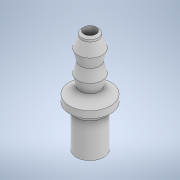
# Autodesk Inventor part: Thread to Barbed 3-32 inch and 10-32 hole
Saved by Autodesk Inventor 2021 (Build 250183000, 183)
## iProperties
Created: 2020-12-17
Part Number: Thread to Barbed 3-32 inch and 10-32 hole
Material: Generic
Document SubType Name: Modeling
Designer: natha
Density: 1 g/cm^3
Appearance: Default
Author: natha
Autodesk Inventor part; units mm, degrees
ref_plane "YZ Plane" through (0, 0, 0) normal (1, 0, 0) x (0, 1, 0)
ref_plane "XZ Plane" through (0, 0, 0) normal (0, 1, 0) x (-1, 0, 0)
ref_plane "XY Plane" through (0, 0, 0) normal (0, 0, 1) x (1, 0, 0)
sketch "Sketch1" plane through (0, 0, 0) normal (0, 0, 1) x (1, 0, 0)
  line L0 (-2, 0) -> (-2, 5)
  line L1 (-2, 5) -> (-3, 6)
  line L2 (-3, 6) -> (-3, 7)
  line L3 (-3, 7) -> (-1.4, 8)
  line L4 (-0.9, 15) -> (-0.9, 0)
  line L5 (-0.9, 0) -> (-2, 0)
  line L6 (0, 18) -> (0, -3) construction
  line L7 (-3.6, 0) -> (0.6, 0) construction
  line L8 (-0.9, 15) -> (-1.2, 14.7)
  line L9 (-1.2, 14.7) -> (-1.2, 14.4)
  line L10 (-1.2, 14.4) -> (-1.8, 12.8)
  line L11 (-1.8, 12.8) -> (-1.4, 11.2)
  line L12 (-1.4, 11.2) -> (-1.8, 9.6)
  line L13 (-1.8, 9.6) -> (-1.4, 8)
  point P0 (0, 0)
  point P1 (-2, 2.5)
  dimension "d0" = 15
  dimension "d4" = 1
  dimension "d5" = 0.9
  dimension "d6" = 1.8
  dimension "d9" = 5
  dimension "d10" = 1
  dimension "d11" = 1
  dimension "d12" = 2.5
  dimension "d14" = 2
  dimension "d15" = 1.2
  dimension "d16" = 1.8
  dimension "d17" = 3
  dimension "d18" = 45
  dimension "d19" = 0.3
  dimension "d20" = 1.4
  dimension "d21" = 1.4
  dimension "d22" = 1.6
  dimension "d23" = 1.6
  dimension "d24" = 1.6
  constraints: 24 end point, 2 vertical, 1 midpoint, 1 parallel, 1 perpendicular
  measures "d0" distance of L4.start L4.end
  measures "d4" distance of L1.end L2.end
  measures "d5" distance between parallel lines of L6 L4
  measures "d6" distance from line of L6 L10.end
  measures "d9" distance from line of L7 L0.end
  measures "d10" horizontal distance of L0.end L1.end
  measures "d11" vertical distance of L3.end L2.end
  measures "d12" distance from line of point (-2, 2.5) L7
  measures "d14" distance from line of L6 point (-2, 2.5)
  measures "d15" distance between parallel lines of L6 L9
  measures "d16" distance from line of L6 L12.end
  measures "d17" distance between parallel lines of L6 L2
  measures "d18" angle of L6 L8
  measures "d19" distance of L8.end L9.end
  measures "d20" distance from line of L6 L11.end
  measures "d21" distance from line of L6 L3.end
  measures "d22" vertical distance of L10.end L9.end
  measures "d23" vertical distance of L3.end L12.end
  measures "d24" vertical distance of L12.end L11.end
revolve "Revolution1" add sketch "Sketch1" angle 360 about axis through (0, 0, 0) along (0, -1, 0)
body "Solid1"
